Autodesk Fusion 360 part; units mm, degrees
note: some values were not read from the file. Set by a fixed rule: which face or edge a step refers to.
(part 2 of 2)
sketch "Sketch37" plane through (0, 0, 110) normal (0, 0, 1) x (-1, 0, 0)
  line L0 (-75, -41) -> (-55, -41)
  line L1 (-55, -41) -> (-55, -39)
  line L2 (-55, -39) -> (-75, -39)
  line L3 (-75, -39) -> (-75, -41)
  circle A0 centre (-126.1011, -76.2995) radius 1.5
  circle A1 centre (-125.9478, -4.1031) radius 1.5
  line L4 (-145, 15) -> (-145, -95)
  line L5 (-145, -95) -> (-75, -41)
  line L6 (-75, -41) -> (-75, -39)
  line L7 (-75, -39) -> (-145, 15)
  circle A2 centre (-3.8154, -76.5304) radius 1.5
  circle A3 centre (-3.7387, -3.9492) radius 1.5
  line L8 (15, -95) -> (15, 15)
  line L9 (15, 15) -> (-55, -39)
  line L10 (-55, -39) -> (-55, -41)
  line L11 (-55, -41) -> (15, -95)
  circle A4 centre (-126.1011, -76.2995) radius 3
  circle A5 centre (-125.9478, -4.1031) radius 3
  circle A6 centre (-3.7387, -3.9492) radius 3
  circle A7 centre (-3.8154, -76.5304) radius 3
  dimension "d262" = 6
  dimension "d263" = 6
  dimension "d264" = 6
  dimension "d265" = 6
  constraint concentric A0 A4
  constraint concentric A1 A5
  constraint concentric A3 A6
  constraint concentric A2 A7
  measures "d262" diameter of A4
  measures "d263" diameter of A5
  measures "d264" diameter of A6
  measures "d265" diameter of A7
extrude "Extrude43" cut sketch "Sketch37" against normal blind 22 contours A4 | A5 | A6 | A7 bodies 4
sketch "Sketch38" plane through (0, 0, 75) normal (0, 0, 1) x (-1, 0, 0)
  circle A0 centre (-3.8154, -76.5304) radius 1.5
  circle A1 centre (-126.1011, -76.2995) radius 1.5
  circle A2 centre (-3.7387, -3.9492) radius 1.5
  circle A3 centre (-125.9478, -4.1031) radius 1.5
  line L0 (-2, -9) -> (-2, -71)
  line L1 (-9, -71) -> (-9, -78)
  line L2 (-9, -78) -> (-121, -78)
  line L3 (-121, -78) -> (-121, -71)
  line L4 (-128, -71) -> (-128, -9)
  line L5 (-121, -2) -> (-9, -2)
  line L6 (-130, -80) -> (0, -80)
  line L7 (0, -80) -> (0, 0)
  line L8 (0, 0) -> (-130, 0)
  line L9 (-130, 0) -> (-130, -80)
  line L10 (-2, -30.2383) -> (-2, -50)
  line L11 (0, -50) -> (0, -40)
  line L12 (0, -50) -> (-2, -50)
  line L13 (0, -40) -> (-2, -40)
  line L14 (0, -50) -> (0, -40)
  line L15 (-2, -40) -> (-2, -50)
  line L16 (-2, -71) -> (-9, -71)
  line L17 (-121, -71) -> (-128, -71)
  line L18 (-128, -9) -> (-121, -9)
  line L19 (-121, -9) -> (-121, -2)
  line L20 (-9, -2) -> (-9, -9)
  line L21 (-9, -9) -> (-2, -9)
  constraint coincident L0 L10.start
  constraint coincident L0 L10.end
  constraint parallel L0 L10
  constraint coincident L7 L11.start
  constraint midpoint L7 L11.end
  constraint parallel L7 L11
  constraint perpendicular L10 L12
  constraint midpoint L0 L13.end
extrude "Extrude44" add sketch "Sketch38" along normal blind 5 contours L0 L7 L10 L11 L12 L13 L14 L15 bodies 1 2
sketch "Sketch39" plane through (0, 0, 75) normal (0, 0, -1) x (1, 0, 0)
  circle A0 centre (3.8154, -76.5304) radius 1.5
  circle A1 centre (126.1011, -76.2995) radius 1.5
  circle A2 centre (3.7387, -3.9492) radius 1.5
  circle A3 centre (125.9478, -4.1031) radius 1.5
  line L0 (-25, -105) -> (155, -105)
  line L1 (155, -105) -> (155, 25)
  line L2 (155, 25) -> (-25, 25)
  line L3 (-25, 25) -> (-25, -105)
  line L4 (2, -30.2383) -> (2, -50)
  line L5 (0, -40) -> (2, -40)
  line L6 (0, -50) -> (0, -40)
  line L7 (0, -50) -> (2, -50)
  line L8 (2, -40) -> (2, -50)
  line L9 (-0.5, -50.5) -> (2.5, -50.5)
  line L10 (2.5, -39.5) -> (2.5, -50.5)
  line L11 (-0.5, -39.5) -> (2.5, -39.5)
  line L12 (-0.5, -50.5) -> (-0.5, -39.5)
  dimension "d270" = 0.5
  constraint coincident L5.end L8.start
  constraint coincident L4.end L7.end
extrude "Extrude45" cut sketch "Sketch39" against normal blind 8 contours L4 L5 L6 L7 L8 | L9 L10 L11 L12 bodies 4
sketch "Sketch40" plane through (0, 0, 40) normal (0, 0, 1) x (-1, 0, 0)
  line L0 (-30, -13) -> (-30, -77)
  line L1 (-30, -77) -> (-3, -77)
  line L2 (-3, -77) -> (-3, -3)
  line L3 (-3, -3) -> (-127, -3)
  line L4 (-127, -3) -> (-127, -13)
  line L5 (-127, -13) -> (-30, -13)
  line L6 (-100, -10) -> (-100, -3)
  line L7 (-100, -10) -> (-98, -10)
  line L8 (-100, -10) -> (-102, -10)
  line L9 (-102, -10) -> (-102, -3)
  line L10 (-98, -10) -> (-98, -3)
  dimension "d273" = 2
  dimension "d274" = 2
  constraint coincident L3 L6.end
  constraint perpendicular L3 L6
  constraint perpendicular L6 L7
  constraint perpendicular L6 L8
  constraint coincident L3 L9.end
  constraint perpendicular L3 L9
  constraint coincident L3 L10.end
  constraint perpendicular L7 L10
  measures "d273" distance of L6.start L7.end
  measures "d274" distance of L6.start L8.end
move_body "Move5" bodies 2 to x (1, 0, 0) y (0, 1, 0) z (0, 0, 1) at (140, 0, -30)
sketch "Sketch42" plane through (0, 0, 10) normal (0, 0, 1) x (-1, 0, 0)
  line L0 (-170, -13) -> (-170, -77)
  line L1 (-170, -77) -> (-143, -77)
  line L2 (-143, -77) -> (-143, -3)
  line L3 (-143, -3) -> (-267, -3)
  line L4 (-267, -3) -> (-267, -13)
  line L5 (-267, -13) -> (-170, -13)
  line L6 (-155.0348, -57.6879) -> (-163.0348, -57.6879)
  line L7 (-163.0348, -57.6879) -> (-163.0348, -69.6879)
  line L8 (-163.0348, -69.6879) -> (-155.0348, -69.6879)
  line L9 (-155.0348, -69.6879) -> (-155.0348, -57.6879)
  dimension "d302" = 8
  dimension "d303" = 12
  constraint horizontal L6
  constraint vertical L7
  constraint horizontal L8
  constraint vertical L9
  measures "d302" distance of L7 L9
  measures "d303" distance of L6 L8
extrude "Extrude48" cut sketch "Sketch42" against normal blind 7 contours L6 L7 L8 L9 bodies 2
sketch "Sketch43" plane through (0, 0, 10) normal (0, 0, 1) x (-1, 0, 0)
  line L0 (-163.0348, -57.6879) -> (-155.0348, -57.6879)
  line L1 (-155.0348, -57.6879) -> (-155.0348, -69.6879)
  line L2 (-155.0348, -69.6879) -> (-163.0348, -69.6879)
  line L3 (-163.0348, -69.6879) -> (-163.0348, -57.6879)
  line L4 (-170, -13) -> (-170, -77)
  line L5 (-170, -77) -> (-143, -77)
  line L6 (-143, -77) -> (-143, -3)
  line L7 (-143, -3) -> (-267, -3)
  line L8 (-267, -3) -> (-267, -13)
  line L9 (-267, -13) -> (-170, -13)
  line L10 (-160.038, -3) -> (-160.038, -11.8021)
  line L11 (-160.038, -11.8021) -> (-250, -11.8021)
  line L12 (-250, -11.8021) -> (-250, -3)
  constraint coincident L7 L10.start
  constraint perpendicular L7 L10
  constraint perpendicular L10 L11
  constraint coincident L7 L12.end
  constraint perpendicular L7 L12
extrude "Extrude49" cut sketch "Sketch43" against normal blind 8 contours L7 L10 L11 L12 bodies 2
sketch "Sketch44" plane through (0, 0, 0) normal (0, 1, 0) x (-1, 0, 0)
  line L0 (-66, 50.6042) -> (-66, 65.6042)
  line L1 (-66, 65.6042) -> (-40, 65.6042)
  line L2 (-40, 65.6042) -> (-40, 50.6042)
  line L3 (-40, 50.6042) -> (-66, 50.6042)
  line L4 (-67.5, 70.1042) -> (-67.5, 38.1042)
  line L5 (-67.5, 38.1042) -> (-38.5, 38.1042)
  line L6 (-38.5, 38.1042) -> (-38.5, 70.1042)
  line L7 (-38.5, 70.1042) -> (-67.5, 70.1042)
  circle A0 centre (-64.5797, 35.2573) radius 2
  circle A1 centre (-41.5797, 35.2573) radius 2
  dimension "d289" = 4
  dimension "d290" = 4
  dimension "d291" = 23
  measures "d289" diameter of A0
  measures "d290" diameter of A1
  measures "d291" horizontal distance of A0.centre A1.centre
sketch "Sketch45" plane through (0, -6, 0) normal (0, -1, 0) x (1, 0, 0)
  line L0 (38.5, 42.1042) -> (67.5, 42.1042)
  line L1 (67.5, 42.1042) -> (67.5, 66.1042)
  line L2 (67.5, 66.1042) -> (38.5, 66.1042)
  line L3 (38.5, 66.1042) -> (38.5, 42.1042)
  line L4 (66, 50.6042) -> (40, 50.6042)
  line L5 (40, 50.6042) -> (40, 65.6042)
  line L6 (40, 65.6042) -> (66, 65.6042)
  line L7 (66, 65.6042) -> (66, 50.6042)
  line L8 (38.5, 42.1042) -> (38.5, 36.1042)
  line L9 (38.5, 36.1042) -> (67.5, 36.1042)
  line L10 (67.5, 36.1042) -> (67.5, 42.1042)
  line L11 (67.5, 42.1042) -> (38.5, 42.1042)
  circle A0 centre (64.5797, 35.2573) radius 3
  circle A1 centre (41.5797, 35.2573) radius 3
  dimension "d296" = 6
  dimension "d297" = 6
  measures "d296" diameter of A0
  measures "d297" diameter of A1
sketch "Sketch46" plane through (0, 0, 0) normal (0, -1, 0) x (1, 0, 0)
  line L0 (38.5, 72.1042) -> (67.5, 72.1042)
  line L1 (67.5, 72.1042) -> (67.5, 70.1042)
  line L2 (67.5, 70.1042) -> (67.5, 38.1042)
  line L3 (67.5, 38.1042) -> (67.5, 36.1042)
  line L4 (67.5, 36.1042) -> (38.5, 36.1042)
  line L5 (38.5, 36.1042) -> (38.5, 38.1042)
  line L6 (38.5, 38.1042) -> (38.5, 70.1042)
  line L7 (38.5, 70.1042) -> (38.5, 72.1042)
  line L8 (80, 72.0884) -> (98.5, 72.0884)
  line L9 (98.5, 72.0884) -> (98.5, 70.0884)
  line L10 (98.5, 70.0884) -> (98.5, 51.5884)
  line L11 (98.5, 51.5884) -> (98.5, 49.5884)
  line L12 (98.5, 49.5884) -> (80, 49.5884)
  line L13 (80, 49.5884) -> (80, 51.5884)
  line L14 (80, 51.5884) -> (80, 70.0884)
  line L15 (80, 70.0884) -> (80, 72.0884)
  line L16 (130, 75) -> (0, 75)
  line L17 (0, 75) -> (0, 0)
  line L18 (0, 0) -> (130, 0)
  line L19 (130, 0) -> (130, 75)
  line L20 (126.26, 10) -> (3.76, 10)
  line L21 (3.76, 10) -> (3.76, 14.5)
  line L22 (3.76, 14.5) -> (15.01, 14.5)
  line L23 (15.01, 14.5) -> (15.01, 26)
  line L24 (15.01, 26) -> (34.01, 26)
  line L25 (34.01, 26) -> (34.01, 14.5)
  line L26 (34.01, 14.5) -> (42.01, 14.5)
  line L27 (42.01, 14.5) -> (42.01, 26)
  line L28 (42.01, 26) -> (61.01, 26)
  line L29 (61.01, 26) -> (61.01, 14.5)
  line L30 (61.01, 14.5) -> (69.01, 14.5)
  line L31 (69.01, 14.5) -> (69.01, 26)
  line L32 (69.01, 26) -> (88.01, 26)
  line L33 (88.01, 26) -> (88.01, 14.5)
  line L34 (88.01, 14.5) -> (96.01, 14.5)
  line L35 (96.01, 14.5) -> (96.01, 26)
  line L36 (96.01, 26) -> (115.01, 26)
  line L37 (115.01, 26) -> (115.01, 14.5)
  line L38 (115.01, 14.5) -> (126.26, 14.5)
  line L39 (126.26, 14.5) -> (126.26, 10)
extrude "Extrude52" add sketch "Sketch46" against normal blind 2 contours L20 L21 L22 L23 L24 L25 L26 L27 L28 L29 L30 L31 L32 L33 L34 L35 L36 L37 L38 L39 bodies 1
move_body "Move6" bodies 2 to x (1, 0, 0) y (0, 1, 0) z (0, 0, 1) at (-140, 0, 30)
sketch "Sketch47" plane through (0, 0, 110) normal (0, 0, 1) x (-1, 0, 0)
  line L0 (-75, -41) -> (-55, -41)
  line L1 (-55, -41) -> (-55, -39)
  line L2 (-55, -39) -> (-75, -39)
  line L3 (-75, -39) -> (-75, -41)
  circle A0 centre (-30, -40) radius 3.4
  dimension "d304" = 6.8
  measures "d304" diameter of A0
extrude "Extrude53" cut sketch "Sketch47" against normal blind 35 contours A0 bodies 4
sketch "Sketch48" plane through (0, 0, 75) normal (0, 0, -1) x (1, 0, 0)
  circle A0 centre (30, -40) radius 3.4
  line L0 (2.5, -39.5) -> (2.5, -50.5)
  line L1 (2.5, -50.5) -> (-0.5, -50.5)
  line L2 (-0.5, -50.5) -> (-0.5, -39.5)
  line L3 (-0.5, -39.5) -> (2.5, -39.5)
  circle A1 centre (3.8154, -76.5304) radius 1.5
  circle A2 centre (126.1011, -76.2995) radius 1.5
  circle A3 centre (3.7387, -3.9492) radius 1.5
  circle A4 centre (125.9478, -4.1031) radius 1.5
  line L4 (-25, -105) -> (155, -105)
  line L5 (155, -105) -> (155, 25)
  line L6 (155, 25) -> (-25, 25)
  line L7 (-25, 25) -> (-25, -105)
  line L8 (45, -25) -> (15, -25)
  line L9 (15, -25) -> (15, -55)
  line L10 (15, -55) -> (45, -55)
  line L11 (45, -55) -> (45, -25)
  line L12 (45, -25) -> (15, -55) construction
  line L13 (15, -25) -> (45, -55) construction
  point P0 (30, -40)
  dimension "d311" = 30
  constraint horizontal L8
  constraint perpendicular L8 L9
  constraint parallel L8 L10
  constraint parallel L9 L11
  constraint coincident L12 P0
  constraint coincident L13 P0
  constraint coincident P0 A0.centre
  measures "d311" distance of L9 L11
extrude "Extrude54" cut sketch "Sketch48" against normal blind 20 contours L8 L9 L10 L11 bodies 4
fillet "Fillet4" radius 10 4 edges at (30, 55, 95) (30, 25, 95) (15, 40, 95) (45, 40, 95) on bodies 4
sketch "Sketch49" plane through (0, 0, 110) normal (0, 0, 1) x (-1, 0, 0)
  line L0 (-75, -41) -> (-55, -41)
  line L1 (-55, -41) -> (-55, -39)
  line L2 (-55, -39) -> (-75, -39)
  line L3 (-75, -39) -> (-75, -41)
  circle A0 centre (-30, -40) radius 3.4
  circle A1 centre (-3.8154, -76.5304) radius 3
  circle A2 centre (-3.7387, -3.9492) radius 3
  line L4 (15, -95) -> (15, 15)
  line L5 (15, 15) -> (-55, -39)
  line L6 (-55, -39) -> (-55, -41)
  line L7 (-55, -41) -> (15, -95)
  line L8 (-30.9585, -44.7541) -> (-26.3621, -43.2071)
  line L9 (-26.3621, -43.2071) -> (-25.4036, -38.453)
  line L10 (-25.4036, -38.453) -> (-29.0415, -35.2459)
  line L11 (-29.0415, -35.2459) -> (-33.6379, -36.7929)
  line L12 (-33.6379, -36.7929) -> (-34.5964, -41.547)
  line L13 (-34.5964, -41.547) -> (-30.9585, -44.7541)
  line L14 (-30.9585, -44.7541) -> (-8.2776, -44.7541) construction
  point P0 (-30, -40)
  dimension "d317" = 8.4
  constraint horizontal L14
  constraint coincident P0 A0.centre
  measures "d317" distance of L9 L12
extrude "Extrude56" cut sketch "Sketch49" against normal blind 12 contours L8 L9 L10 L11 L12 L13 bodies 4
sketch "Sketch50" plane through (0, 0, 0) normal (0, 0, -1) x (1, 0, 0)
  line L0 (130, 0) -> (0, 0)
  line L1 (0, 0) -> (0, -80)
  line L2 (0, -80) -> (4.76, -80)
  line L3 (4.76, -80) -> (4.76, -93)
  line L4 (4.76, -93) -> (125.26, -93)
  line L5 (125.26, -93) -> (125.26, -80)
  line L6 (125.26, -80) -> (130, -80)
  line L7 (130, -80) -> (130, 0)
  line L8 (130, 0) -> (140, 0)
  line L9 (130, 0) -> (150, 0)
  line L10 (150, 0) -> (150, -10)
  line L11 (150, -10) -> (130, -10)
  line L12 (130, -80) -> (150, -80)
  line L13 (150, -80) -> (150, -70)
  line L14 (150, -70) -> (130, -70)
  line L15 (0, -80) -> (-20, -80)
  line L16 (-20, -80) -> (-20, -70)
  line L17 (-20, -70) -> (0, -70)
  line L18 (0, 0) -> (-20, 0)
  line L19 (-20, 0) -> (-20, -10)
  line L20 (-20, -10) -> (0, -10)
  arc A0 (130, -50) -> (130, -30) centre (130, -40) ccw
  arc A1 (130, -46) -> (130, -34) centre (130, -40) ccw
  arc A2 (0, -30) -> (0, -50) centre (0, -40) ccw
  arc A3 (0, -34) -> (0, -46) centre (0, -40) ccw
  dimension "d318" = -4
  dimension "d319" = -4
  constraint coincident L0.start L7.end
  constraint perpendicular L7 L8
  constraint perpendicular L7 L9
  constraint perpendicular L9 L10
  constraint coincident L7 L11.end
  constraint perpendicular L7 L11
  constraint coincident L6.end L7.start
  constraint perpendicular L7 L12
  constraint perpendicular L12 L13
  constraint coincident L7 L14.end
  constraint perpendicular L7 L14
  constraint coincident L1.end L2.start
  constraint perpendicular L1 L15
  constraint perpendicular L15 L16
  constraint coincident L1 L17.end
  constraint perpendicular L1 L17
  constraint coincident L0.end L1.start
  constraint perpendicular L1 L18
  constraint perpendicular L18 L19
  constraint coincident L1 L20.end
  constraint perpendicular L1 L20
  constraint coincident L7 A0.start
  constraint coincident L7 A0.end
  constraint coincident L1 A2.end
  constraint coincident L1 A2.start
extrude "Extrude57" add sketch "Sketch50" against normal blind 5 contours L7 L8 L9 L10 L11 | L1 L18 L19 L20 | L7 A0 A1 | L1 A2 A3 | L7 L12 L13 L14 | L1 L15 L16 L17 bodies 1 2 4
sketch "Sketch51" plane through (0, 0, 5) normal (0, 0, 1) x (-1, 0, 0)
  line L0 (-150, 0) -> (-150, -10)
  line L1 (-150, -10) -> (-130, -10)
  line L2 (-130, -10) -> (-130, 0)
  line L3 (-130, 0) -> (-150, 0)
  line L4 (-150, -80) -> (-130, -80)
  line L5 (-130, -80) -> (-130, -70)
  line L6 (-130, -70) -> (-150, -70)
  line L7 (-150, -70) -> (-150, -80)
  line L8 (-130, -5) -> (-150, -5)
  line L9 (-140, 0) -> (-140, -10)
  line L10 (-140, -10) -> (-145, -10)
  line L11 (-145, -10) -> (-145, 0)
  line L12 (-145, 0) -> (-145, -80)
  line L13 (-150, -75) -> (-130, -75)
  circle A0 centre (-145, -5) radius 2
  circle A1 centre (-145, -75) radius 2
  circle A2 centre (-145, -5) radius 3.5
  circle A3 centre (-145, -75) radius 3.5
  dimension "d322" = 5
  dimension "d323" = 4
  dimension "d324" = 4
  dimension "d327" = 7
  dimension "d328" = 7
  constraint midpoint L2 L8.start
  constraint midpoint L0 L8.end
  constraint midpoint L3 L9.start
  constraint perpendicular L8 L9
  constraint coincident L1 L10.end
  constraint perpendicular L9 L10
  constraint coincident L3 L11.end
  constraint perpendicular L3 L11
  constraint coincident L4 L12.end
  constraint perpendicular L4 L12
  constraint midpoint L7 L13.start
  constraint midpoint L5 L13.end
  constraint midpoint L11 A0.centre
  constraint coincident L13 A1.centre
  constraint coincident L12 A1.centre
  constraint concentric A0 A2
  constraint concentric A1 A3
  measures "d322" distance of L9.end L10.end
  measures "d323" diameter of A0
  measures "d324" diameter of A1
  measures "d327" diameter of A2
  measures "d328" diameter of A3
extrude "Extrude58" cut sketch "Sketch51" against normal blind 6 contours L8 L11 L12 A0 | L8 L11 L12 A0 | L8 L11 L12 A0 | L8 L11 L12 A0 | L12 L13 A1 | L12 L13 A1 | L12 L13 A1 | L12 L13 A1 bodies 1
extrude "Extrude59" cut sketch "Sketch51" against normal blind 3 contours L8 L11 L12 A0 A2 | L8 L11 L12 A0 A2 | L8 L11 L12 A0 A2 | L8 L11 L12 A0 A2 | L12 L13 A1 A3 | L12 L13 A1 A3 | L12 L13 A1 A3 | L12 L13 A1 A3 bodies 1
sketch "Sketch52" plane through (0, 0, 5) normal (0, 0, 1) x (-1, 0, 0)
  line L0 (20, -80) -> (20, -70)
  line L1 (20, -70) -> (0, -70)
  line L2 (0, -70) -> (0, -80)
  line L3 (0, -80) -> (20, -80)
  line L4 (20, 0) -> (0, 0)
  line L5 (0, 0) -> (0, -10)
  line L6 (0, -10) -> (20, -10)
  line L7 (20, -10) -> (20, 0)
  line L8 (20, -75) -> (0, -75)
  line L9 (20, -5) -> (0, -5)
  line L10 (20, 0) -> (15, 0)
  line L11 (15, 0) -> (15, -80)
  circle A0 centre (15, -75) radius 2
  circle A1 centre (15, -5) radius 2
  circle A2 centre (15, -5) radius 3.5
  circle A3 centre (15, -75) radius 3.5
  dimension "d331" = 5
  dimension "d332" = 4
  dimension "d333" = 4
  dimension "d334" = 7
  dimension "d335" = 7
  constraint midpoint L0 L8.start
  constraint midpoint L2 L8.end
  constraint midpoint L7 L9.start
  constraint midpoint L5 L9.end
  constraint coincident L4.start L7.end
  constraint perpendicular L5 L10
  constraint coincident L3 L11.end
  constraint perpendicular L3 L11
  constraint coincident L11 A0.centre
  constraint coincident L8 A0.centre
  constraint coincident L11 A1.centre
  constraint coincident L9 A1.centre
  constraint concentric A1 A2
  constraint concentric A0 A3
  measures "d331" distance of L4.start L10.end
  measures "d332" diameter of A0
  measures "d333" diameter of A1
  measures "d334" diameter of A2
  measures "d335" diameter of A3
extrude "Extrude60" cut sketch "Sketch52" against normal blind 5 contours L8 L11 A0 | L8 L11 A0 | L8 L11 A0 | L8 L11 A0 | L9 L11 A1 | L9 L11 A1 | L9 L11 A1 | L9 L11 A1 bodies 1
extrude "Extrude61" cut sketch "Sketch52" against normal blind 3 contours L8 L11 A0 A3 | L8 L11 A0 A3 | L8 L11 A0 A3 | L8 L11 A0 A3 | L9 L11 A1 A2 | L9 L11 A1 A2 | L9 L11 A1 A2 | L9 L11 A1 A2 bodies 1
move_body "Move7" bodies 2 to x (1, 0, 0) y (0, 1, 0) z (0, 0, 1) at (-170, 0, -30)
move_body "Move8" bodies 4 to x (1, 0, 0) y (0, 1, 0) z (0, 0, 1) at (-340, 0, -70)
fillet "Fillet5" radius 3 2 edges at (140, 40, 5) (-10, 40, 5) on bodies 1
extrude "Extrude62" cut 1 faces at (47.0764, 15.9708, 10) along direction (0, 0, -1) blind 1 on bodies 1 bodies 1
sketch "Sketch53" plane through (0, 0, 9) normal (0, 0, 1) x (-1, 0, 0)
  line L0 (-2, -2) -> (-128, -2)
  line L1 (-128, -2) -> (-128, -78)
  line L2 (-128, -78) -> (-125.26, -78)
  line L3 (-125.26, -78) -> (-125.26, -80)
  line L4 (-125.26, -80) -> (-125.26, -93)
  line L5 (-125.26, -93) -> (-4.76, -93)
  line L6 (-4.76, -93) -> (-4.76, -80)
  line L7 (-4.76, -80) -> (-4.76, -78)
  line L8 (-4.76, -78) -> (-2, -78)
  line L9 (-2, -78) -> (-2, -2)
  circle A0 centre (-9.51, -44.9344) radius 2
  circle A1 centre (-120.51, -45.0177) radius 2
  line L10 (-125.26, -93) -> (-125.26, -95)
  line L11 (-125.26, -95) -> (-4.76, -95)
  line L12 (-4.76, -95) -> (-4.76, -93)
  dimension "d345" = 2
  constraint coincident L4.end L5.start
  constraint perpendicular L5 L10
  constraint perpendicular L6 L11
  constraint coincident L5.end L6.start
  constraint perpendicular L5 L12
  measures "d345" distance of L4.end L10.end
extrude "Extrude63" add sketch "Sketch53" along normal blind 2 and the other way blind 9 contours L5 L10 L11 L12 bodies 1
sketch "Sketch54" plane through (0, 2, 0) normal (0, 1, 0) x (-1, 0, 0)
  line L0 (-2, 9) -> (-2, 21)
  line L1 (-2, 21) -> (-12, 21)
  line L2 (-12, 21) -> (-12, 33)
  line L3 (-12, 33) -> (-2, 33)
  line L4 (-2, 33) -> (-2, 68)
  line L5 (-9, 68) -> (-9, 75)
  line L6 (-9, 75) -> (-121, 75)
  line L7 (-121, 75) -> (-121, 68)
  line L8 (-128, 68) -> (-128, 33)
  line L9 (-128, 33) -> (-118, 33)
  line L10 (-118, 33) -> (-118, 21)
  line L11 (-118, 21) -> (-128, 21)
  line L12 (-128, 21) -> (-128, 9)
  line L13 (-128, 9) -> (-2, 9)
  line L14 (-38.5, 38.1042) -> (-67.5, 38.1042)
  line L15 (-67.5, 38.1042) -> (-67.5, 70.1042)
  line L16 (-67.5, 70.1042) -> (-38.5, 70.1042)
  line L17 (-38.5, 70.1042) -> (-38.5, 38.1042)
  line L18 (-80, 51.5884) -> (-98.5, 51.5884)
  line L19 (-98.5, 51.5884) -> (-98.5, 70.0884)
  line L20 (-98.5, 70.0884) -> (-80, 70.0884)
  line L21 (-80, 70.0884) -> (-80, 51.5884)
  line L22 (-68, 37.6042) -> (-68, 70.6042)
  line L23 (-68, 70.6042) -> (-38, 70.6042)
  line L24 (-38, 70.6042) -> (-38, 37.6042)
  line L25 (-38, 37.6042) -> (-68, 37.6042)
  line L26 (-38, 37.6042) -> (-35, 37.6042)
  line L27 (-35, 37.6042) -> (-35, 70.6042)
  line L28 (-35, 70.6042) -> (-38, 70.6042)
  line L29 (-68, 37.6042) -> (-71, 37.6042)
  line L30 (-71, 37.6042) -> (-71, 70.6042)
  line L31 (-71, 70.6042) -> (-68, 70.6042)
  line L32 (-35, 37.6042) -> (-71, 37.6042)
  line L33 (-35, 37.6042) -> (-35, 34.6042)
  line L34 (-35, 34.6042) -> (-71, 34.6042)
  line L35 (-71, 34.6042) -> (-71, 37.6042)
  line L36 (-2, 68) -> (-9, 68)
  line L37 (-121, 68) -> (-128, 68)
  dimension "d350" = -0.5
  dimension "d351" = 3
  dimension "d352" = 3
  dimension "d353" = 3
  constraint perpendicular L24 L26
  constraint perpendicular L26 L27
  constraint perpendicular L24 L28
  constraint perpendicular L22 L29
  constraint perpendicular L23 L30
  constraint perpendicular L22 L31
  constraint perpendicular L26 L33
  constraint perpendicular L30 L34
  constraint perpendicular L29 L35
  measures "d351" distance of L24.end L26.end
  measures "d352" distance of L22.start L29.end
  measures "d353" distance of L26.end L33.end
extrude "Extrude64" add sketch "Sketch54" along normal blind 7 contours L22 L29 L30 L31 L32 | L25 L26 L29 L32 L33 L34 L35 | L24 L26 L27 L28 L32 bodies 1
sketch "Sketch55" plane through (0, 9, 0) normal (0, 1, 0) x (-1, 0, 0)
  line L0 (-35, 34.6042) -> (-35, 70.6042)
  line L1 (-35, 70.6042) -> (-38, 70.6042)
  line L2 (-38, 70.6042) -> (-38, 37.6042)
  line L3 (-38, 37.6042) -> (-68, 37.6042)
  line L4 (-68, 37.6042) -> (-68, 70.6042)
  line L5 (-68, 70.6042) -> (-71, 70.6042)
  line L6 (-71, 70.6042) -> (-71, 34.6042)
  line L7 (-71, 34.6042) -> (-35, 34.6042)
  line L8 (-38, 70.6042) -> (-40, 70.6042)
  line L9 (-40, 70.6042) -> (-40, 40)
  line L10 (-68, 70.6042) -> (-66, 70.6042)
  line L11 (-66, 70.6042) -> (-66, 40)
  line L12 (-66, 40) -> (-40, 40)
  dimension "d356" = 2
  constraint coincident L1.end L2.start
  constraint perpendicular L2 L8
  constraint perpendicular L3 L9
  constraint coincident L4.end L5.start
  constraint perpendicular L4 L10
  constraint perpendicular L10 L11
  constraint perpendicular L9 L12
  measures "d356" distance of L4.end L10.end
extrude "Extrude65" add sketch "Sketch55" against normal blind 2.4 contours L2 L3 L4 L8 L9 L10 L11 L12 bodies 1
extrude "Extrude66" add 1 faces at (57.3333, 0, 42.2709) along direction (0, 1, 0) blind 2 on bodies 1 bodies 1
sketch "Sketch56" plane through (0, 2, 0) normal (0, 1, 0) x (-1, 0, 0)
  line L0 (-66, 50.6042) -> (-66, 65.6042)
  line L1 (-66, 65.6042) -> (-40, 65.6042)
  line L2 (-40, 65.6042) -> (-40, 50.6042)
  line L3 (-40, 50.6042) -> (-66, 50.6042)
  line L4 (-35, 34.6042) -> (-71, 34.6042)
  line L5 (-71, 34.6042) -> (-71, 70.6042)
  line L6 (-71, 70.6042) -> (-68, 70.6042)
  line L7 (-68, 70.6042) -> (-68, 37.6042)
  line L8 (-68, 37.6042) -> (-38, 37.6042)
  line L9 (-38, 37.6042) -> (-38, 70.6042)
  line L10 (-38, 70.6042) -> (-35, 70.6042)
  line L11 (-35, 70.6042) -> (-35, 34.6042)
  line L12 (-2, 9) -> (-2, 21)
  line L13 (-2, 21) -> (-12, 21)
  line L14 (-12, 21) -> (-12, 33)
  line L15 (-12, 33) -> (-2, 33)
  line L16 (-2, 33) -> (-2, 68)
  line L17 (-9, 68) -> (-9, 75)
  line L18 (-9, 75) -> (-121, 75)
  line L19 (-121, 75) -> (-121, 68)
  line L20 (-128, 68) -> (-128, 33)
  line L21 (-128, 33) -> (-118, 33)
  line L22 (-118, 33) -> (-118, 21)
  line L23 (-118, 21) -> (-128, 21)
  line L24 (-128, 21) -> (-128, 9)
  line L25 (-128, 9) -> (-2, 9)
  line L26 (-80, 51.5884) -> (-98.5, 51.5884)
  line L27 (-98.5, 51.5884) -> (-98.5, 70.0884)
  line L28 (-98.5, 70.0884) -> (-80, 70.0884)
  line L29 (-80, 70.0884) -> (-80, 51.5884)
  line L30 (-99, 51.0884) -> (-99, 70.5884)
  line L31 (-99, 70.5884) -> (-79.5, 70.5884)
  line L32 (-79.5, 70.5884) -> (-79.5, 51.0884)
  line L33 (-79.5, 51.0884) -> (-99, 51.0884)
  line L34 (-79.5, 51.0884) -> (-76.5, 51.0884)
  line L35 (-76.5, 51.0884) -> (-76.5, 70.5884)
  line L36 (-76.5, 70.5884) -> (-79.5, 70.5884)
  line L37 (-99, 70.5884) -> (-102, 70.5884)
  line L38 (-102, 70.5884) -> (-102, 51.0884)
  line L39 (-102, 51.0884) -> (-99, 51.0884)
  line L40 (-76.5, 51.0884) -> (-76.5, 48.0884)
  line L41 (-76.5, 48.0884) -> (-102, 48.0884)
  line L42 (-102, 48.0884) -> (-102, 51.0884)
  line L43 (-2, 68) -> (-9, 68)
  line L44 (-121, 68) -> (-128, 68)
  dimension "d361" = -0.5
  dimension "d362" = 3
  dimension "d363" = 3
  dimension "d364" = 3
  constraint perpendicular L32 L34
  constraint perpendicular L31 L35
  constraint perpendicular L32 L36
  constraint perpendicular L30 L37
  constraint perpendicular L33 L38
  constraint perpendicular L30 L39
  constraint perpendicular L33 L40
  constraint perpendicular L38 L41
  constraint perpendicular L39 L42
  measures "d362" distance of L32.end L34.end
  measures "d363" distance of L30.end L37.end
  measures "d364" distance of L34.end L40.end
extrude "Extrude67" add sketch "Sketch56" along normal blind 7 contours L30 L37 L38 L39 | L33 L34 L39 L40 L41 L42 | L32 L34 L35 L36 bodies 1
sketch "Sketch57" plane through (0, 9, 0) normal (0, 1, 0) x (-1, 0, 0)
  line L0 (-76.5, 48.0884) -> (-76.5, 70.5884)
  line L1 (-76.5, 70.5884) -> (-79.5, 70.5884)
  line L2 (-79.5, 70.5884) -> (-79.5, 51.0884)
  line L3 (-79.5, 51.0884) -> (-99, 51.0884)
  line L4 (-99, 51.0884) -> (-99, 70.5884)
  line L5 (-99, 70.5884) -> (-102, 70.5884)
  line L6 (-102, 70.5884) -> (-102, 48.0884)
  line L7 (-102, 48.0884) -> (-76.5, 48.0884)
  line L8 (-79.5, 70.5884) -> (-81.5, 70.5884)
  line L9 (-81.5, 70.5884) -> (-81.5, 53.0884)
  line L10 (-99, 70.5884) -> (-97, 70.5884)
  line L11 (-97, 70.5884) -> (-97, 53.0884)
  line L12 (-97, 53.0884) -> (-81.5, 53.0884)
  dimension "d367" = 2
  dimension "d368" = 17.5
  dimension "d369" = 2
  constraint coincident L1.end L2.start
  constraint perpendicular L2 L8
  constraint perpendicular L3 L9
  constraint coincident L4.end L5.start
  constraint perpendicular L4 L10
  constraint perpendicular L10 L11
  constraint perpendicular L9 L12
  measures "d367" distance of L1.end L8.end
  measures "d368" distance of L8.end L9.end
  measures "d369" distance of L4.end L10.end
extrude "Extrude68" add sketch "Sketch57" against normal blind 4 contours L2 L3 L4 L8 L9 L10 L11 L12 bodies 1
extrude "Extrude69" add 1 faces at (96.4167, 0, 59.8384) along direction (0, 1, 0) blind 2 on bodies 1 bodies 1
sketch "Sketch58" plane through (0, 2, 0) normal (0, 1, 0) x (-1, 0, 0)
  line L0 (-92.25, 63.8384) -> (-86.25, 63.8384)
  line L1 (-86.25, 63.8384) -> (-86.25, 57.8384)
  line L2 (-86.25, 57.8384) -> (-92.25, 57.8384)
  line L3 (-92.25, 57.8384) -> (-92.25, 63.8384)
  line L4 (-76.5, 48.0884) -> (-102, 48.0884)
  line L5 (-102, 48.0884) -> (-102, 70.5884)
  line L6 (-102, 70.5884) -> (-99, 70.5884)
  line L7 (-99, 70.5884) -> (-99, 51.0884)
  line L8 (-99, 51.0884) -> (-79.5, 51.0884)
  line L9 (-79.5, 51.0884) -> (-79.5, 70.5884)
  line L10 (-79.5, 70.5884) -> (-76.5, 70.5884)
  line L11 (-76.5, 70.5884) -> (-76.5, 48.0884)
  line L12 (-66, 50.6042) -> (-66, 65.6042)
  line L13 (-66, 65.6042) -> (-40, 65.6042)
  line L14 (-40, 65.6042) -> (-40, 50.6042)
  line L15 (-40, 50.6042) -> (-66, 50.6042)
  line L16 (-35, 34.6042) -> (-71, 34.6042)
  line L17 (-71, 34.6042) -> (-71, 70.6042)
  line L18 (-71, 70.6042) -> (-68, 70.6042)
  line L19 (-68, 70.6042) -> (-68, 37.6042)
  line L20 (-68, 37.6042) -> (-38, 37.6042)
  line L21 (-38, 37.6042) -> (-38, 70.6042)
  line L22 (-38, 70.6042) -> (-35, 70.6042)
  line L23 (-35, 70.6042) -> (-35, 34.6042)
  line L24 (-2, 9) -> (-2, 21)
  line L25 (-2, 21) -> (-12, 21)
  line L26 (-12, 21) -> (-12, 33)
  line L27 (-12, 33) -> (-2, 33)
  line L28 (-2, 33) -> (-2, 68)
  line L29 (-9, 68) -> (-9, 75)
  line L30 (-9, 75) -> (-121, 75)
  line L31 (-121, 75) -> (-121, 68)
  line L32 (-128, 68) -> (-128, 33)
  line L33 (-128, 33) -> (-118, 33)
  line L34 (-118, 33) -> (-118, 21)
  line L35 (-118, 21) -> (-128, 21)
  line L36 (-128, 21) -> (-128, 9)
  line L37 (-128, 9) -> (-2, 9)
  line L38 (-94.25, 55.8384) -> (-94.25, 65.8384)
  line L39 (-94.25, 65.8384) -> (-84.25, 65.8384)
  line L40 (-84.25, 65.8384) -> (-84.25, 55.8384)
  line L41 (-84.25, 55.8384) -> (-94.25, 55.8384)
  line L42 (-84.25, 65.8384) -> (-84.25, 75)
  line L43 (-94.25, 65.8384) -> (-94.25, 75)
  line L44 (-2, 68) -> (-9, 68)
  line L45 (-121, 68) -> (-128, 68)
  dimension "d374" = -2
  constraint coincident L30 L42.end
  constraint perpendicular L30 L42
  constraint coincident L30 L43.end
  constraint perpendicular L30 L43
extrude "Extrude70" cut sketch "Sketch58" against normal blind 1 contours L30 L39 L42 L43 | L38 L39 L40 L41 bodies 1
sketch "Sketch59" plane through (0, 2, 0) normal (0, 1, 0) x (-1, 0, 0)
  line L0 (-84.25, 75) -> (-84.25, 55.8384)
  line L1 (-84.25, 55.8384) -> (-94.25, 55.8384)
  line L2 (-94.25, 55.8384) -> (-94.25, 75)
  line L3 (-94.25, 75) -> (-121, 75)
  line L4 (-121, 75) -> (-121, 68)
  line L5 (-128, 68) -> (-128, 33)
  line L6 (-128, 33) -> (-118, 33)
  line L7 (-118, 33) -> (-118, 21)
  line L8 (-118, 21) -> (-128, 21)
  line L9 (-128, 21) -> (-128, 9)
  line L10 (-128, 9) -> (-2, 9)
  line L11 (-2, 9) -> (-2, 21)
  line L12 (-2, 21) -> (-12, 21)
  line L13 (-12, 21) -> (-12, 33)
  line L14 (-12, 33) -> (-2, 33)
  line L15 (-2, 33) -> (-2, 68)
  line L16 (-9, 68) -> (-9, 75)
  line L17 (-9, 75) -> (-84.25, 75)
  line L18 (-35, 34.6042) -> (-71, 34.6042)
  line L19 (-71, 34.6042) -> (-71, 70.6042)
  line L20 (-71, 70.6042) -> (-68, 70.6042)
  line L21 (-68, 70.6042) -> (-68, 37.6042)
  line L22 (-68, 37.6042) -> (-38, 37.6042)
  line L23 (-38, 37.6042) -> (-38, 70.6042)
  line L24 (-38, 70.6042) -> (-35, 70.6042)
  line L25 (-35, 70.6042) -> (-35, 34.6042)
  line L26 (-66, 50.6042) -> (-66, 65.6042)
  line L27 (-66, 65.6042) -> (-40, 65.6042)
  line L28 (-40, 65.6042) -> (-40, 50.6042)
  line L29 (-40, 50.6042) -> (-66, 50.6042)
  line L30 (-76.5, 48.0884) -> (-102, 48.0884)
  line L31 (-102, 48.0884) -> (-102, 70.5884)
  line L32 (-102, 70.5884) -> (-99, 70.5884)
  line L33 (-99, 70.5884) -> (-99, 51.0884)
  line L34 (-99, 51.0884) -> (-79.5, 51.0884)
  line L35 (-79.5, 51.0884) -> (-79.5, 70.5884)
  line L36 (-79.5, 70.5884) -> (-76.5, 70.5884)
  line L37 (-76.5, 70.5884) -> (-76.5, 48.0884)
  line L38 (-67, 49.6042) -> (-67, 66.6042)
  line L39 (-67, 66.6042) -> (-39, 66.6042)
  line L40 (-39, 66.6042) -> (-39, 49.6042)
  line L41 (-39, 49.6042) -> (-67, 49.6042)
  line L42 (-39, 66.6042) -> (-39, 75)
  line L43 (-67, 66.6042) -> (-67, 75)
  line L44 (-121, 68) -> (-128, 68)
  line L45 (-2, 68) -> (-9, 68)
  dimension "d377" = -1
  constraint coincident L17 L42.end
  constraint perpendicular L17 L42
  constraint coincident L17 L43.end
  constraint perpendicular L17 L43
extrude "Extrude71" cut sketch "Sketch59" against normal blind 1 contours L17 L39 L42 L43 | L38 L39 L40 L41 bodies 1
move_body "Move9" bodies 2 to x (1, 0, 0) y (0, 1, 0) z (0, 0, 1) at (170, 0, 30)
move_body "Move10" bodies 2 to x (1, 0, 0) y (0, 1, 0) z (0, 0, 1) at (-160, 0, -30)
sketch "Sketch60" plane through (0, 0, 8) normal (0, 0, 1) x (-1, 0, 0)
  circle A0 centre (36.8, -16.8) radius 1.6
  circle A1 centre (126.2, -73.2) radius 1.6
  circle A2 centre (126.2, -16.8) radius 1.6
  line L0 (33, -13) -> (33, -77)
  line L1 (33, -77) -> (130, -77)
  line L2 (130, -77) -> (130, -13)
  line L3 (130, -13) -> (33, -13)
  line L4 (50, -11.8021) -> (50, -3)
  line L5 (50, -3) -> (33, -3)
  line L6 (33, -3) -> (33, -13)
  line L7 (33, -13) -> (130, -13)
  line L8 (130, -13) -> (130, -77)
  line L9 (130, -77) -> (157, -77)
  line L10 (157, -77) -> (157, -3)
  line L11 (157, -3) -> (139.962, -3)
  line L12 (139.962, -3) -> (139.962, -11.8021)
  line L13 (139.962, -11.8021) -> (50, -11.8021)
  line L14 (136.9652, -57.6879) -> (144.9652, -57.6879)
  line L15 (144.9652, -57.6879) -> (144.9652, -69.6879)
  line L16 (144.9652, -69.6879) -> (136.9652, -69.6879)
  line L17 (136.9652, -69.6879) -> (136.9652, -57.6879)
  line L18 (130, -13) -> (130, -11.8021)
  line L19 (50, -11.8021) -> (50, -13)
  line L20 (130, -13) -> (139.962, -13)
  line L21 (139.962, -13) -> (139.962, -11.8021)
  constraint coincident L2.end L3.start
  constraint coincident L13 L18.end
  constraint perpendicular L13 L18
  constraint coincident L4.start L13.end
  constraint coincident L7 L19.end
  constraint perpendicular L7 L19
  constraint perpendicular L12 L20
  constraint coincident L12.end L13.start
  constraint perpendicular L13 L21
extrude "Extrude72" cut sketch "Sketch60" along normal blind -5 and the other way blind -2 contours L3 L7 L13 L18 L19 | L13 L18 L20 L21 bodies 2
move_body "Move11" bodies 2 to x (1, 0, 0) y (0, 1, 0) z (0, 0, 1) at (160, 0, 30)
extrude "Extrude73" add 1 faces at (99, 3, 57.5884) along direction (-1, 0, 0) blind 0.62 on bodies 1 bodies 1
extrude "Extrude74" add 1 faces at (79.5, 3, 64.0884) along direction (1, 0, 0) blind 0.62 on bodies 1 bodies 1
extrude "Extrude75" add 1 faces at (38, 5.0667, 59.6042) along direction (1, 0, 0) blind 0.3 on bodies 1 bodies 1
extrude "Extrude76" add 1 faces at (68, 3.5333, 59.6042) along direction (-1, 0, 0) blind 0.3 on bodies 1 bodies 1
move_body "Move12" bodies 2 to x (1, 0, 0) y (0, 1, 0) z (0, 0, 1) at (-158, 0, -32)
chamfer "Chamfer15" distance 2 angle 45 24 edges at (47.75, 80, 49) (40, 80, 45) (55.5, 80, 45) (60.5, 80, 45) (68.25, 80, 49) (76, 80, 45) (81, 80, 45) (88.75, 80, 49) (96.5, 80, 45) (101.5, 80, 45) (109.25, 80, 49) (117, 80, 45) (103.75, 80, 55) (109.25, 80, 58.5) (114.75, 80, 55) (83.25, 80, 55) (88.75, 80, 58.5) (94.25, 80, 55) (73.75, 80, 55) (68.25, 80, 58.5) (62.75, 80, 55) (53.25, 80, 55) (47.75, 80, 58.5) (42.25, 80, 55) on bodies 1
chamfer "Chamfer16" distance 2 angle 45 19 edges at (24.51, 80, 25) (16.01, 80, 19.25) (43.01, 80, 19.25) (51.51, 80, 25) (70.01, 80, 19.25) (78.51, 80, 25) (97.01, 80, 19.25) (105.51, 80, 25) (114.01, 80, 19.25) (87.01, 80, 19.25) (119.635, 80, 13.5) (92.01, 80, 13.5) (65.01, 80, 13.5) (38.01, 80, 13.5) (60.01, 80, 19.25) (33.01, 80, 19.25) (10.385, 80, 13.5) (125.26, 80, 11.25) (4.76, 80, 11.25) on bodies 1
sketch "Sketch61" plane through (0, 0, 33) normal (0, 0, 1) x (-1, 0, 0)
  line L0 (-118, -78) -> (-118, -66)
  line L1 (-118, -66) -> (-128, -66)
  line L2 (-128, -66) -> (-128, -78)
  line L3 (-128, -78) -> (-118, -78)
  line L4 (-118, -66) -> (-115, -66)
  line L5 (-115, -66) -> (-115, -78)
  line L6 (-115, -78) -> (-118, -78)
  line L7 (-12, -78) -> (-2, -78)
  line L8 (-2, -78) -> (-2, -66)
  line L9 (-2, -66) -> (-12, -66)
  line L10 (-12, -66) -> (-12, -78)
  line L11 (-2, -2) -> (-12, -2)
  line L12 (-12, -2) -> (-12, -14)
  line L13 (-12, -14) -> (-2, -14)
  line L14 (-2, -14) -> (-2, -2)
  line L15 (-118, -14) -> (-118, -2)
  line L16 (-118, -2) -> (-128, -2)
  line L17 (-128, -2) -> (-128, -14)
  line L18 (-128, -14) -> (-118, -14)
  line L19 (-12, -66) -> (-15, -66)
  line L20 (-15, -66) -> (-15, -78)
  line L21 (-15, -78) -> (-12, -78)
  line L22 (-12, -14) -> (-15, -14)
  line L23 (-15, -14) -> (-15, -2)
  line L24 (-15, -2) -> (-12, -2)
  line L25 (-118, -14) -> (-115, -14)
  line L26 (-115, -14) -> (-115, -2)
  line L27 (-115, -2) -> (-118, -2)
  dimension "d396" = 3
  dimension "d397" = 3
  dimension "d398" = 3
  dimension "d399" = 3
  constraint coincident L0.end L1.start
  constraint perpendicular L0 L4
  constraint perpendicular L3 L5
  constraint coincident L0.start L3.end
  constraint perpendicular L0 L6
  constraint coincident L9.end L10.start
  constraint perpendicular L10 L19
  constraint perpendicular L7 L20
  constraint coincident L7.start L10.end
  constraint perpendicular L10 L21
  constraint coincident L12.end L13.start
  constraint perpendicular L12 L22
  constraint perpendicular L11 L23
  constraint coincident L11.end L12.start
  constraint perpendicular L12 L24
  constraint coincident L15.start L18.end
  constraint perpendicular L15 L25
  constraint perpendicular L16 L26
  constraint coincident L15.end L16.start
  constraint perpendicular L15 L27
  measures "d396" distance of L0.end L4.end
  measures "d397" distance of L9.end L19.end
  measures "d398" distance of L12.end L22.end
  measures "d399" distance of L15.start L25.end
extrude "Extrude77" add sketch "Sketch61" against normal blind 12 contours L0 L4 L5 L6 | L10 L19 L20 L21 | L12 L22 L23 L24 | L15 L25 L26 L27 bodies 1
move_body "Move13" bodies 2 to x (1, 0, 0) y (0, 1, 0) z (0, 0, 1) at (158, 0, 33)
sketch "Sketch62" plane through (0, 0, 41) normal (0, 0, 1) x (-1, 0, 0)
  line L0 (-110, -13) -> (-110, -3)
  line L1 (-110, -3) -> (-127, -3)
  line L2 (-127, -3) -> (-127, -13)
  line L3 (-127, -13) -> (-110, -13)
  line L4 (-115, -2) -> (-128, -2)
  line L5 (-128, -2) -> (-128, -14)
  line L6 (-128, -14) -> (-115, -14)
  line L7 (-115, -14) -> (-115, -2)
  line L8 (-2, -2) -> (-15, -2)
  line L9 (-15, -2) -> (-15, -14)
  line L10 (-15, -14) -> (-2, -14)
  line L11 (-2, -14) -> (-2, -2)
  line L12 (-15, -78) -> (-2, -78)
  line L13 (-2, -78) -> (-2, -66)
  line L14 (-2, -66) -> (-15, -66)
  line L15 (-15, -66) -> (-15, -78)
  line L16 (-115, -66) -> (-128, -66)
  line L17 (-128, -66) -> (-128, -78)
  line L18 (-128, -78) -> (-115, -78)
  line L19 (-115, -78) -> (-115, -66)
  circle A0 centre (-118.1089, -7.4281) radius 1.5
  circle A1 centre (-11.8631, -6.602) radius 1.5
  circle A2 centre (-12.1707, -71.8391) radius 1.5
  circle A3 centre (-117.89, -71.7808) radius 1.5
  dimension "d402" = 3
  dimension "d403" = 3
  dimension "d404" = 3
  dimension "d405" = 3
  measures "d402" diameter of A0
  measures "d403" diameter of A1
  measures "d404" diameter of A2
  measures "d405" diameter of A3
extrude "Extrude78" cut sketch "Sketch62" against normal blind 19 contours A0 | A1 | A2 | A3 bodies 1 2
sketch "Sketch63" plane through (0, 0, 9) normal (0, 0, 1) x (-1, 0, 0)
  line L0 (-2, -2) -> (-128, -2)
  line L1 (-128, -2) -> (-128, -78)
  line L2 (-128, -78) -> (-125.26, -78)
  line L3 (-125.26, -78) -> (-127.26, -80)
  line L4 (-127.26, -80) -> (-125.26, -80)
  line L5 (-125.26, -80) -> (-125.26, -93)
  line L6 (-125.26, -93) -> (-4.76, -93)
  line L7 (-4.76, -93) -> (-4.76, -80)
  line L8 (-4.76, -80) -> (-2.76, -80)
  line L9 (-2.76, -80) -> (-4.76, -78)
  line L10 (-4.76, -78) -> (-2, -78)
  line L11 (-2, -78) -> (-2, -2)
  circle A0 centre (-9.51, -44.9344) radius 2
  circle A1 centre (-120.51, -45.0177) radius 2
  circle A2 centre (-8.26, -89.5) radius 1.5
  circle A3 centre (-121.76, -89.5) radius 1.5
  dimension "d409" = 3
  dimension "d410" = 3.5
  dimension "d411" = 3.5
  dimension "d412" = 3
  dimension "d413" = 3.5
  dimension "d414" = 3.5
  measures "d409" diameter of A2
  measures "d410" distance of L6 A2.centre
  measures "d411" distance of L7 A2.centre
  measures "d412" diameter of A3
  measures "d413" distance of L6 A3.centre
  measures "d414" distance of L5 A3.centre
extrude "Extrude79" cut sketch "Sketch63" against normal blind 9 contours A2 | A3 bodies 1
chamfer "Chamfer17" distance 7 angle 45 4 edges at (124.5, 71, 68) (5.5, 71, 68) (124.5, 9, 68) (5.5, 9, 68) on bodies 1
chamfer "Chamfer18" distance 12 angle 45 4 edges at (121.5, 66, 21) (8.5, 66, 21) (121.5, 14, 21) (8.5, 14, 21) on bodies 1
chamfer "Chamfer19" distance 7 angle 45 1 edges at (89.25, 9, 48.0884) on bodies 1
chamfer "Chamfer20" distance 7 angle 45 1 edges at (53, 9, 34.6042) on bodies 1
move_body "Move14" bodies 4 to x (1, 0, 0) y (0, 1, 0) z (0, 0, 1) at (340, 0, 60)
move_body "Move15" bodies 4 to x (1, 0, 0) y (0, 1, 0) z (0, 0, 1) at (0, 0, 10)
named bodies: "Smart Garden Base", "Smart Garden Platform", "Smart Garden Lid"
